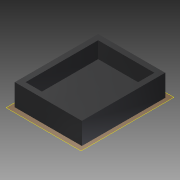
# Autodesk Inventor part: InlayUnten
Saved by Autodesk Inventor 2014 (Build 180170000, 170)
## iProperties
Created: 2016-09-06
Part Number: InlayUnten
Material: Kautschuk
Document SubType Name: Modeling
Designer: cem
Density: 1 g/cm^3
Appearance: Gummi - schwarz - Version 1.1
Author: cem
Autodesk Inventor part; units mm, degrees
ref_plane "YZ Plane" through (0, 0, 0) normal (1, 0, 0) x (0, 1, 0)
ref_plane "XZ Plane" through (0, 0, 0) normal (0, 1, 0) x (-1, 0, 0)
ref_plane "XY Plane" through (0, 0, 0) normal (0, 0, 1) x (1, 0, 0)
ref_plane "Arbeitsebene1" through (0, 0, 0) normal (0, 0, 1) x (1, 0, 0)
sketch "Skizze1" plane through (0, 0, 0) normal (0, 0, 1) x (1, 0, 0)
  line L0 (-33.9, 46.4) -> (-33.9, -46.4) projected
  line L1 (-33.9, -46.4) -> (33.9, -46.4) projected
  line L2 (33.9, -46.4) -> (33.9, 46.4) projected
  line L3 (33.9, 46.4) -> (-33.9, 46.4) projected
  line L4 (-33.4, 45.9) -> (-33.4, -45.9)
  line L5 (-33.4, -45.9) -> (33.4, -45.9)
  line L6 (33.4, -45.9) -> (33.4, 45.9)
  line L7 (33.4, 45.9) -> (-33.4, 45.9)
  point P0 (0, 0)
  dimension "d0" = 0.5
  constraints: 8 end point, 3 other
  measures "d0" distance between parallel lines of L3 L7
extrude "Extrusion1" add sketch "Skizze1" along normal blind 5 contours L7 L6 L5 L4
sketch "Skizze2" plane through (0, 0, 5) normal (0, 0, 1) x (1, 0, 0)
  line L0 (-33.4, 45.9) -> (-33.4, -45.9) projected
  line L1 (-33.4, -45.9) -> (33.4, -45.9) projected
  line L2 (33.4, -45.9) -> (33.4, 45.9) projected
  line L3 (33.4, 45.9) -> (-33.4, 45.9) projected
  line L4 (-28.4, 40.9) -> (-28.4, -40.9)
  line L5 (-28.4, -40.9) -> (28.4, -40.9)
  line L6 (28.4, -40.9) -> (28.4, 40.9)
  line L7 (28.4, 40.9) -> (-28.4, 40.9)
  point P0 (0, 0)
  dimension "d3" = 5
  constraints: 8 end point, 3 other
  measures "d3" distance between parallel lines of L4 L0
extrude "Extrusion2" add sketch "Skizze2" along normal blind 15
